Microcontroller Pin_v2 (Autodesk Fusion 360 design; units mm, degrees)
Autodesk Fusion 360 part; units mm, degrees
sketch "Sketch1" plane through (0, 0, 0) normal (0, 0, 1) x (1, 0, 0)
  circle A0 centre (0, 0) radius 0.975
  dimension "d1" = 1.95
  constraint coincident A0.centre origin
  measures "d1" diameter of A0
extrude "Extrude1" add sketch "Sketch1" along normal blind 6
sketch "Sketch2" plane through (0, 0, 0) normal (0, 0, -1) x (1, 0, 0)
  circle A0 centre (0, 0) radius 0.975
  circle A1 centre (0, 0) radius 1.75
  dimension "d4" = 3.5
  constraint concentric A0 A1
  measures "d4" diameter of A1
extrude "Extrude2" add sketch "Sketch2" along normal blind 1.5 contours A0 | A1
extrude "Extrude3" cut 1 faces at (-0.5048, -0.8743, -1.5) along direction (0, 0, 1) blind 0.5
equation "d4 = ( 1.75 * 2 ) * 1 mm"
